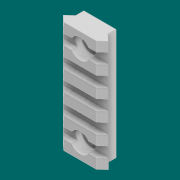
# Autodesk Inventor part: Picatinny2Hole
Saved by Autodesk Inventor 2020.4 (Build 244396010, 396A)
## iProperties
Created: 2022-09-13
Part Number: Picatinny2Hole
Material: Generic
Document SubType Name: Modeling
Designer: Val
Density: 1 g/cm^3
Appearance: Default
Author: Val
Autodesk Inventor part; units mm, degrees
ref_plane "YZ Plane" through (0, 0, 0) normal (1, 0, 0) x (0, 1, 0)
ref_plane "XZ Plane" through (0, 0, 0) normal (0, 1, 0) x (-1, 0, 0)
ref_plane "XY Plane" through (0, 0, 0) normal (0, 0, 1) x (1, 0, 0)
sketch "Base" plane through (0, 0, 0) normal (0, 0, 1) x (1, 0, 0)
  circle A0 centre (0, 0) radius 1.9844
  line L0 (0, 0) -> (0, 39.37) construction
  circle A1 centre (0, 39.37) radius 1.9844
  line L1 (-7.8169, 49.657) -> (7.8169, 49.657)
  line L2 (7.8169, 49.657) -> (7.8169, -10.287)
  line L3 (7.8169, -10.287) -> (-7.8169, -10.287)
  line L4 (-7.8169, -10.287) -> (-7.8169, 49.657)
  line L5 (0, 0) -> (0, -10.287) construction
  line L6 (0, 39.37) -> (0, 49.657) construction
  dimension "d0" = 3.9688
  dimension "d1" = 39.37
  dimension "d2" = 15.6337
  dimension "d3" = 59.944
  dimension "d4" = 10.287
  dimension "d5" = 10.287
  constraints: 14 end point, 2 centre point, 2 coincident, 2 midpoint, 2 parallel, 2 perpendicular, 1 equal radius, 1 horizontal, 1 vertical
  measures "d0" diameter of A0
  measures "d1" distance of L0.start L0.end
  measures "d2" distance of L2.end L3.end
  measures "d3" distance of L3.end L1.start
  measures "d4" distance of L0.start L5.end
  measures "d5" distance from line of L1 L0.end
extrude "BaseFeature" add sketch "Base" along normal blind 4.064
sketch "Profile" plane through (-7.8169, -10.287, 0) normal (0, -1, 0) x (1, 0, 0)
  line L0 (0, 4.064) -> (15.6337, 4.064) projected
  line L1 (15.7353, 6.858) -> (18.7833, 6.858) construction
  line L2 (15.6337, 4.064) -> (15.7353, 4.064)
  line L3 (15.7353, 4.064) -> (15.7353, 6.858) construction
  line L4 (15.7353, 4.064) -> (18.7833, 6.858)
  line L5 (18.7833, 6.858) -> (15.7353, 9.652)
  line L6 (15.7353, 6.858) -> (15.7353, 9.652) construction
  line L7 (7.8169, 4.064) -> (7.8169, 9.652) construction
  line L8 (7.8169, 9.652) -> (15.7353, 9.652)
  line L9 (0, 4.064) -> (-0.1016, 4.064)
  line L10 (-0.1016, 4.064) -> (-3.1496, 6.858)
  line L11 (-3.1496, 6.858) -> (-0.1016, 9.652)
  line L12 (7.8169, 9.652) -> (-0.1016, 9.652)
  point P0 (7.8169, 0)
  dimension "d9" = 3.048
  dimension "d10" = 0.1016
  dimension "d11" = 2.794
  dimension "d12" = 42.51
  dimension "d13" = 42.51
  constraints: 25 end point, 3 symmetric about line, 2 perpendicular, 2 vertical, 1 collinear, 1 horizontal, 1 midpoint
  measures "d9" distance of L1.start L1.end
  measures "d10" distance of L0.end L2.end
  measures "d11" distance of L2.end L1.start
  measures "d12" angle of L1 L4
  measures "d13" angle of L1 L5
extrude "ProfileFeature" add sketch "Profile" against normal up to surface (59.944 mm away)
sketch "Ridges" plane through (-7.9185, -10.287, 9.652) normal (0, 0, 1) x (1, 0, 0)
  line L0 (18.8849, 0) -> (18.8849, 59.944)
  line L1 (-3.048, 52.2224) -> (18.8849, 52.2224)
  line L2 (18.8849, 52.2224) -> (18.8849, 47.0916)
  line L3 (18.8849, 47.0916) -> (-3.048, 47.0916)
  line L4 (-3.048, 47.0916) -> (-3.048, 52.2224)
  line L5 (-3.048, 42.3926) -> (18.8849, 42.3926)
  line L6 (18.8849, 42.3926) -> (18.8849, 37.2618)
  line L7 (18.8849, 37.2618) -> (-3.048, 37.2618)
  line L8 (-3.048, 37.2618) -> (-3.048, 42.3926)
  line L9 (-3.048, 0) -> (-3.048, 59.944)
  line L10 (-3.048, 32.5628) -> (18.8849, 32.5628)
  line L11 (18.8849, 32.5628) -> (18.8849, 27.432)
  line L12 (18.8849, 27.432) -> (-3.048, 27.432)
  line L13 (-3.048, 27.432) -> (-3.048, 32.5628)
  line L14 (-3.048, 29.972) -> (18.8849, 29.972) construction
  line L15 (-3.048, 56.9214) -> (18.8849, 56.9214) construction
  line L16 (15.8369, 59.944) -> (0, 59.944)
  line L17 (-3.048, 22.733) -> (18.8849, 22.733)
  line L18 (18.8849, 22.733) -> (18.8849, 17.6022)
  line L19 (18.8849, 17.6022) -> (-3.048, 17.6022)
  line L20 (-3.048, 17.6022) -> (-3.048, 22.733)
  line L21 (-3.048, 12.9032) -> (18.8849, 12.9032)
  line L22 (18.8849, 12.9032) -> (18.8849, 7.7724)
  line L23 (18.8849, 7.7724) -> (-3.048, 7.7724)
  line L24 (-3.048, 7.7724) -> (-3.048, 12.9032)
  line L25 (-3.048, 49.657) -> (18.8849, 49.657) construction
  circle A0 centre (7.9185, 49.657) radius 1.9844 construction
  point P0 (7.9185, 10.287)
  point P1 (-3.048, 7.7724)
  point P2 (-3.048, 17.6022)
  point P3 (-3.048, 27.432)
  dimension "d16" = 4.699
  dimension "d17" = 4.699
  dimension "d18" = 5.1308
  dimension "d19" = 5.1308
  dimension "d20" = 5.1308
  dimension "d21" = 4.699
  dimension "d23" = 4.699
  dimension "d24" = 5.1308
  dimension "d25" = 4.699
  dimension "d26" = 5.1308
  constraints: 46 end point, 10 parallel, 6 horizontal, 5 perpendicular, 4 midpoint, 4 point on line, 1 coincident, 8 other
  measures "d16" distance between parallel lines of L5 L3
  measures "d17" distance between parallel lines of L10 L7
  measures "d18" distance between parallel lines of L7 L5
  measures "d19" distance of L3.end L1.start
  measures "d20" distance of L12.end L10.start
  measures "d21" distance between parallel lines of L1 L15
  measures "d23" distance between parallel lines of L17 L12
  measures "d24" distance between parallel lines of L19 L17
  measures "d25" distance between parallel lines of L21 L19
  measures "d26" distance between parallel lines of L23 L21
extrude "RidgesFeature" cut sketch "Ridges" against normal up to surface (2.794 mm away) contours L23 L9 L21 L0 | L19 L9 L17 L0 | L12 L9 L10 L0 | L7 L8 L5 L0 | L3 L4 L1 L0
sketch "MountHoles" plane through (-10.9664, 41.9354, 6.858) normal (0, 0, 1) x (1, 0, 0)
  circle A0 centre (10.9664, -41.9354) radius 1.9844 projected
  circle A1 centre (10.9664, -2.5654) radius 1.9844 projected
  circle A2 centre (10.9664, -41.9354) radius 4.826
  circle A3 centre (10.9664, -2.5654) radius 4.826
  dimension "d29" = 9.652
  dimension "d30" = 9.652
  constraints: 2 centre point, 2 coincident
  measures "d29" diameter of A2
  measures "d30" diameter of A3
extrude "MountHolesFeature" cut sketch "MountHoles" against normal up to surface (2.794 mm away) contours A0 | A1 | A2 | A3
extrude "CountersinksFeature" cut sketch "MountHoles" along normal through all contours A0 | A1 | A2 | A3
sketch "Trim" plane through (-7.9185, 32.1056, 9.652) normal (0, 0, 1) x (1, 0, 0)
  line L0 (-3.048, 0) -> (-3.048, 4.699) projected
  line L1 (-3.048, 17.5514) -> (0, 17.5514) projected
  line L2 (-3.048, 17.5514) -> (18.8849, 17.5514)
  line L3 (18.8849, 17.5514) -> (18.8849, 14.5288)
  line L4 (18.8849, 14.5288) -> (-3.048, 14.5288)
  line L5 (-3.048, 14.5288) -> (-3.048, 17.5514)
  line L6 (0, 9.8298) -> (3.8308, 9.8298) projected
  line L7 (18.8849, 9.8298) -> (18.8849, 17.5514) projected
  line L8 (-3.048, -42.3926) -> (0, -42.3926) projected
  line L9 (-3.048, -42.3926) -> (18.8849, -42.3926)
  line L10 (18.8849, -42.3926) -> (18.8849, -39.37)
  line L11 (18.8849, -39.37) -> (-3.048, -39.37)
  line L12 (-3.048, -39.37) -> (-3.048, -42.3926)
  line L13 (18.8849, -42.3926) -> (18.8849, -34.6202) projected
  point P0 (7.9185, -32.1056)
  dimension "d35" = 4.699
  dimension "d36" = 4.699
  constraints: 16 end point, 4 parallel, 3 collinear, 2 horizontal, 2 perpendicular
  measures "d35" distance of L0.start L0.end
  measures "d36" distance between parallel lines of L4 L6
extrude "TrimFeature" cut sketch "Trim" against normal through all
equation "\"d4\" = d5"
equation "\"d13\" = d12"
equation "\"d16\" = d21"
equation "\"d17\" = d21"
equation "\"d19\" = d18"
equation "\"d20\" = d18"
equation "\"d23\" = d21"
equation "\"d24\" = d20"
equation "\"d25\" = d21"
equation "\"d26\" = d20"
equation "\"d36\" = d35"
body "Solid1"
